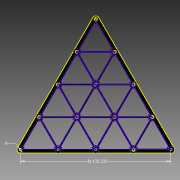
# Autodesk Inventor part: g16-bezel
Saved by Autodesk Inventor 2013 (Build 170138000, 138)
## iProperties
Created: 2013-03-21
Part Number: g16-bezel
Material: Acrylic
Document SubType Name: Modeling
Designer: TechShop Member
Density: 1 g/cm^3
d2: 6.000 mm
d5: 3.000 mm
Bolt_HeadDiameter: 6.000 mm
Bolt_HoleDiameter: 3.000 mm
LayerThickness: 2.750 mm
Pixel_BorderWidth: 1.000 mm
Pixel_Stride: 33.333 mm
Base_SideWidth: 133.332 mm
d24: 6.000 mm
d4: 0.00 deg
Author: TechShop Member
Autodesk Inventor part; units mm, degrees
(part 1 of 2)
ref_plane "YZ Plane" through (0, 0, 0) normal (1, 0, 0) x (0, 1, 0)
ref_plane "XZ Plane" through (0, 0, 0) normal (0, 1, 0) x (-1, 0, 0)
ref_plane "XY Plane" through (0, 0, 0) normal (0, 0, 1) x (1, 0, 0)
sketch "Triangle Hole Template" plane through (0, 0, 0) normal (0, 0, 1) x (1, 0, 0)
  line L0 (-99.9974, -57.7156) -> (-66.6644, -57.7156) construction
  line L1 (-66.6644, -57.7156) -> (-83.3309, -86.5829) construction
  line L2 (-83.3309, -86.5829) -> (-99.9974, -57.7156) construction
  line L3 (-99.1314, -58.2156) -> (-67.5304, -58.2156) construction
  line L4 (-67.5304, -58.2156) -> (-83.3309, -85.5829) construction
  line L5 (-83.3309, -85.5829) -> (-99.1314, -58.2156) construction
  line L6 (-83.3309, -58.2156) -> (-83.3309, -57.7156) construction
  line L7 (-75.4307, -71.8992) -> (-74.9976, -72.1492) construction
  line L8 (-91.2311, -71.8992) -> (-91.6641, -72.1492) construction
  arc A0 (-68.5696, -60.0156) -> (-69.6089, -58.2156) centre (-69.6089, -59.4156) ccw
  arc A1 (-84.3701, -83.7829) -> (-82.2917, -83.7829) centre (-83.3309, -83.1829) ccw
  arc A2 (-97.0529, -58.2156) -> (-98.0921, -60.0156) centre (-97.0529, -59.4156) ccw
  line L9 (-97.0529, -58.2156) -> (-69.6089, -58.2156)
  line L10 (-68.5696, -60.0156) -> (-82.2917, -83.7829)
  line L11 (-84.3701, -83.7829) -> (-98.0921, -60.0156)
  circle A3 centre (-98.4385, -58.6156) radius 0.4 construction
  line L12 (-98.0921, -58.8156) -> (-98.785, -58.4156) construction
  circle A4 centre (-99.9974, -57.7156) radius 3 construction
  line L13 (-83.3309, -57.7156) -> (-83.3309, -57.2156) construction
  line L14 (-98.0921, -58.8156) -> (-97.3993, -59.2156) construction
  point P0 (-85.6081, -66.0431)
  dimension "d24" = 6
  dimension "Pixel_BorderWidth" = 1
  dimension "Pixel_Stride" = 33.333
  measures "Pixel_BorderWidth" distance of L13.end L6.start
  measures "Pixel_Stride" distance of L0.start L0.end
sketch "Triangle Hole Template x16" plane through (0, 0, 0) normal (0, 0, 1) x (1, 0, 0)
  line L0 (-99.9974, -57.7156) -> (-66.6644, -57.7156) construction
  line L1 (-66.6644, -57.7156) -> (-83.3309, -86.5829) construction
  line L2 (-83.3309, -86.5829) -> (-99.9974, -57.7156) construction
  line L3 (-99.1314, -58.2156) -> (-67.5304, -58.2156) construction
  line L4 (-67.5304, -58.2156) -> (-83.3309, -85.5829) construction
  line L5 (-83.3309, -85.5829) -> (-99.1314, -58.2156) construction
  line L6 (-83.3309, -58.2156) -> (-83.3309, -57.7156) construction
  line L7 (-75.4307, -71.8992) -> (-74.9976, -72.1492) construction
  line L8 (-91.2311, -71.8992) -> (-91.6641, -72.1492) construction
  arc A0 (-68.5696, -60.0156) -> (-69.6089, -58.2156) centre (-69.6089, -59.4156) ccw
  arc A1 (-84.3701, -83.7829) -> (-82.2917, -83.7829) centre (-83.3309, -83.1829) ccw
  arc A2 (-97.0529, -58.2156) -> (-98.0921, -60.0156) centre (-97.0529, -59.4156) ccw
  line L9 (-97.0529, -58.2156) -> (-69.6089, -58.2156)
  line L10 (-68.5696, -60.0156) -> (-82.2917, -83.7829)
  line L11 (-84.3701, -83.7829) -> (-98.0921, -60.0156)
  circle A3 centre (-98.4385, -58.6156) radius 0.4 construction
  line L12 (-98.0921, -58.8156) -> (-98.785, -58.4156) construction
  circle A4 centre (-99.9974, -57.7156) radius 3 construction
  line L13 (-83.3309, -57.7156) -> (-83.3309, -57.2156) construction
  line L14 (-98.0921, -58.8156) -> (-97.3993, -59.2156) construction
  line L15 (-83.3309, -86.5829) -> (-49.9979, -86.5829) construction
  line L16 (-49.9979, -86.5829) -> (-66.6644, -115.4501) construction
  line L17 (-66.6644, -115.4501) -> (-83.3309, -86.5829) construction
  line L18 (-82.4649, -87.0829) -> (-50.8639, -87.0829) construction
  line L19 (-50.8639, -87.0829) -> (-66.6644, -114.4501) construction
  line L20 (-66.6644, -114.4501) -> (-82.4649, -87.0829) construction
  line L21 (-66.6644, -87.0829) -> (-66.6644, -86.5829) construction
  line L22 (-58.7642, -100.7665) -> (-58.3311, -101.0165) construction
  line L23 (-74.5646, -100.7665) -> (-74.9976, -101.0165) construction
  arc A5 (-51.9031, -88.8829) -> (-52.9424, -87.0829) centre (-52.9424, -88.2829) ccw
  arc A6 (-67.7036, -112.6501) -> (-65.6252, -112.6501) centre (-66.6644, -112.0501) ccw
  arc A7 (-80.3864, -87.0829) -> (-81.4256, -88.8829) centre (-80.3864, -88.2829) ccw
  line L24 (-80.3864, -87.0829) -> (-52.9424, -87.0829)
  line L25 (-51.9031, -88.8829) -> (-65.6252, -112.6501)
  line L26 (-67.7036, -112.6501) -> (-81.4256, -88.8829)
  circle A8 centre (-81.772, -87.4829) radius 0.4 construction
  line L27 (-81.4256, -87.6829) -> (-82.1185, -87.2829) construction
  circle A9 centre (-83.3309, -86.5829) radius 3 construction
  line L28 (-66.6644, -86.5829) -> (-66.6644, -86.0829) construction
  line L29 (-81.4256, -87.6829) -> (-80.7328, -88.0829) construction
  line L30 (-66.6676, -57.7533) -> (-33.3346, -57.7533) construction
  line L31 (-33.3346, -57.7533) -> (-50.0011, -86.6205) construction
  line L32 (-50.0011, -86.6205) -> (-66.6676, -57.7533) construction
  line L33 (-65.8016, -58.2533) -> (-34.2006, -58.2533) construction
  line L34 (-34.2006, -58.2533) -> (-50.0011, -85.6205) construction
  line L35 (-50.0011, -85.6205) -> (-65.8016, -58.2533) construction
  line L36 (-50.0011, -58.2533) -> (-50.0011, -57.7533) construction
  line L37 (-42.1009, -71.9369) -> (-41.6679, -72.1869) construction
  line L38 (-57.9013, -71.9369) -> (-58.3344, -72.1869) construction
  arc A10 (-35.2399, -60.0533) -> (-36.2791, -58.2533) centre (-36.2791, -59.4533) ccw
  arc A11 (-51.0403, -83.8205) -> (-48.9619, -83.8205) centre (-50.0011, -83.2205) ccw
  arc A12 (-63.7231, -58.2533) -> (-64.7624, -60.0533) centre (-63.7231, -59.4533) ccw
  line L39 (-63.7231, -58.2533) -> (-36.2791, -58.2533)
  line L40 (-35.2399, -60.0533) -> (-48.9619, -83.8205)
  line L41 (-51.0403, -83.8205) -> (-64.7624, -60.0533)
  circle A13 centre (-65.1088, -58.6533) radius 0.4 construction
  line L42 (-64.7624, -58.8533) -> (-65.4552, -58.4533) construction
  circle A14 centre (-66.6676, -57.7533) radius 3 construction
  line L43 (-50.0011, -57.7533) -> (-50.0011, -57.2533) construction
  line L44 (-64.7624, -58.8533) -> (-64.0695, -59.2533) construction
  line L45 (-50.0011, -86.6205) -> (-83.3341, -86.6205) construction
  line L46 (-83.3341, -86.6205) -> (-66.6676, -57.7533) construction
  line L47 (-66.6676, -57.7533) -> (-50.0011, -86.6205) construction
  line L48 (-50.8671, -86.1205) -> (-82.4681, -86.1205) construction
  line L49 (-82.4681, -86.1205) -> (-66.6676, -58.7533) construction
  line L50 (-66.6676, -58.7533) -> (-50.8671, -86.1205) construction
  line L51 (-66.6676, -86.1205) -> (-66.6676, -86.6205) construction
  line L52 (-74.5678, -72.4369) -> (-75.0009, -72.1869) construction
  line L53 (-58.7674, -72.4369) -> (-58.3344, -72.1869) construction
  arc A15 (-81.4289, -84.3205) -> (-80.3896, -86.1205) centre (-80.3896, -84.9205) ccw
  arc A16 (-65.6284, -60.5533) -> (-67.7068, -60.5533) centre (-66.6676, -61.1533) ccw
  arc A17 (-52.9456, -86.1205) -> (-51.9064, -84.3205) centre (-52.9456, -84.9205) ccw
  line L54 (-52.9456, -86.1205) -> (-80.3896, -86.1205)
  line L55 (-81.4289, -84.3205) -> (-67.7068, -60.5533)
  line L56 (-65.6284, -60.5533) -> (-51.9064, -84.3205)
  circle A18 centre (-51.56, -85.7205) radius 0.4 construction
  line L57 (-51.9064, -85.5205) -> (-51.2135, -85.9205) construction
  circle A19 centre (-50.0011, -86.6205) radius 3 construction
  line L58 (-66.6676, -86.6205) -> (-66.6676, -87.1205) construction
  line L59 (-51.9064, -85.5205) -> (-52.5992, -85.1205) construction
  line L60 (-33.3346, -57.7533) -> (-66.6676, -57.7533) construction
  line L61 (-66.6676, -57.7533) -> (-50.0011, -28.886) construction
  line L62 (-50.0011, -28.886) -> (-33.3346, -57.7533) construction
  line L63 (-34.2006, -57.2533) -> (-65.8016, -57.2533) construction
  line L64 (-65.8016, -57.2533) -> (-50.0011, -29.886) construction
  line L65 (-50.0011, -29.886) -> (-34.2006, -57.2533) construction
  line L66 (-50.0011, -57.2533) -> (-50.0011, -57.7533) construction
  line L67 (-57.9013, -43.5697) -> (-58.3344, -43.3197) construction
  line L68 (-42.1009, -43.5697) -> (-41.6679, -43.3197) construction
  arc A20 (-64.7624, -55.4533) -> (-63.7231, -57.2533) centre (-63.7231, -56.0533) ccw
  arc A21 (-48.9619, -31.686) -> (-51.0403, -31.686) centre (-50.0011, -32.286) ccw
  arc A22 (-36.2791, -57.2533) -> (-35.2399, -55.4533) centre (-36.2791, -56.0533) ccw
  line L69 (-36.2791, -57.2533) -> (-63.7231, -57.2533)
  line L70 (-64.7624, -55.4533) -> (-51.0403, -31.686)
  line L71 (-48.9619, -31.686) -> (-35.2399, -55.4533)
  circle A23 centre (-34.8935, -56.8533) radius 0.4 construction
  line L72 (-35.2399, -56.6533) -> (-34.547, -57.0533) construction
  circle A24 centre (-33.3346, -57.7533) radius 3 construction
  line L73 (-50.0011, -57.7533) -> (-50.0011, -58.2533) construction
  line L74 (-35.2399, -56.6533) -> (-35.9327, -56.2533) construction
  line L75 (-66.6676, -57.7156) -> (-100.0006, -57.7156) construction
  line L76 (-100.0006, -57.7156) -> (-83.3341, -28.8484) construction
  line L77 (-83.3341, -28.8484) -> (-66.6676, -57.7156) construction
  line L78 (-67.5336, -57.2156) -> (-99.1346, -57.2156) construction
  line L79 (-99.1346, -57.2156) -> (-83.3341, -29.8484) construction
  line L80 (-83.3341, -29.8484) -> (-67.5336, -57.2156) construction
  line L81 (-83.3341, -57.2156) -> (-83.3341, -57.7156) construction
  line L82 (-91.2343, -43.532) -> (-91.6674, -43.282) construction
  line L83 (-75.4339, -43.532) -> (-75.0009, -43.282) construction
  arc A25 (-98.0954, -55.4156) -> (-97.0561, -57.2156) centre (-97.0561, -56.0156) ccw
  arc A26 (-82.2949, -31.6484) -> (-84.3733, -31.6484) centre (-83.3341, -32.2484) ccw
  arc A27 (-69.6121, -57.2156) -> (-68.5729, -55.4156) centre (-69.6121, -56.0156) ccw
  line L84 (-69.6121, -57.2156) -> (-97.0561, -57.2156)
  line L85 (-98.0954, -55.4156) -> (-84.3733, -31.6484)
  line L86 (-82.2949, -31.6484) -> (-68.5729, -55.4156)
  circle A28 centre (-68.2265, -56.8156) radius 0.4 construction
  line L87 (-68.5729, -56.6156) -> (-67.88, -57.0156) construction
  circle A29 centre (-66.6676, -57.7156) radius 3 construction
  line L88 (-83.3341, -57.7156) -> (-83.3341, -58.2156) construction
  line L89 (-68.5729, -56.6156) -> (-69.2657, -56.2156) construction
  line L90 (-83.3186, -28.8752) -> (-116.6516, -28.8752) construction
  line L91 (-116.6516, -28.8752) -> (-99.9851, -0.008) construction
  line L92 (-99.9851, -0.008) -> (-83.3186, -28.8752) construction
  line L93 (-84.1846, -28.3752) -> (-115.7856, -28.3752) construction
  line L94 (-115.7856, -28.3752) -> (-99.9851, -1.008) construction
  line L95 (-99.9851, -1.008) -> (-84.1846, -28.3752) construction
  line L96 (-99.9851, -28.3752) -> (-99.9851, -28.8752) construction
  line L97 (-107.8853, -14.6916) -> (-108.3184, -14.4416) construction
  line L98 (-92.0849, -14.6916) -> (-91.6519, -14.4416) construction
  arc A30 (-114.7464, -26.5752) -> (-113.7071, -28.3752) centre (-113.7071, -27.1752) ccw
  arc A31 (-98.9459, -2.808) -> (-101.0243, -2.808) centre (-99.9851, -3.408) ccw
  arc A32 (-86.2631, -28.3752) -> (-85.2239, -26.5752) centre (-86.2631, -27.1752) ccw
  line L99 (-86.2631, -28.3752) -> (-113.7071, -28.3752)
  line L100 (-114.7464, -26.5752) -> (-101.0243, -2.808)
  line L101 (-98.9459, -2.808) -> (-85.2239, -26.5752)
  circle A33 centre (-84.8775, -27.9752) radius 0.4 construction
  line L102 (-85.2239, -27.7752) -> (-84.531, -28.1752) construction
  circle A34 centre (-83.3186, -28.8752) radius 3 construction
  line L103 (-99.9851, -28.8752) -> (-99.9851, -29.3752) construction
  line L104 (-85.2239, -27.7752) -> (-85.9167, -27.3752) construction
  line L105 (-50.0011, -28.8484) -> (-83.3341, -28.8484) construction
  line L106 (-83.3341, -28.8484) -> (-66.6676, 0.0188) construction
  line L107 (-66.6676, 0.0188) -> (-50.0011, -28.8484) construction
  line L108 (-50.8671, -28.3484) -> (-82.4681, -28.3484) construction
  line L109 (-82.4681, -28.3484) -> (-66.6676, -0.9812) construction
  line L110 (-66.6676, -0.9812) -> (-50.8671, -28.3484) construction
  line L111 (-66.6676, -28.3484) -> (-66.6676, -28.8484) construction
  line L112 (-74.5678, -14.6648) -> (-75.0009, -14.4148) construction
  line L113 (-58.7674, -14.6648) -> (-58.3344, -14.4148) construction
  arc A35 (-81.4289, -26.5484) -> (-80.3896, -28.3484) centre (-80.3896, -27.1484) ccw
  arc A36 (-65.6284, -2.7812) -> (-67.7068, -2.7812) centre (-66.6676, -3.3812) ccw
  arc A37 (-52.9456, -28.3484) -> (-51.9064, -26.5484) centre (-52.9456, -27.1484) ccw
  line L114 (-52.9456, -28.3484) -> (-80.3896, -28.3484)
  line L115 (-81.4289, -26.5484) -> (-67.7068, -2.7812)
  line L116 (-65.6284, -2.7812) -> (-51.9064, -26.5484)
  circle A38 centre (-51.56, -27.9484) radius 0.4 construction
  line L117 (-51.9064, -27.7484) -> (-51.2135, -28.1484) construction
  circle A39 centre (-50.0011, -28.8484) radius 3 construction
  line L118 (-66.6676, -28.8484) -> (-66.6676, -29.3484) construction
  line L119 (-51.9064, -27.7484) -> (-52.5992, -27.3484) construction
  line L120 (-16.6681, -28.8484) -> (-50.0011, -28.8484) construction
  line L121 (-50.0011, -28.8484) -> (-33.3346, 0.0188) construction
  line L122 (-33.3346, 0.0188) -> (-16.6681, -28.8484) construction
  line L123 (-17.5341, -28.3484) -> (-49.1351, -28.3484) construction
  line L124 (-49.1351, -28.3484) -> (-33.3346, -0.9812) construction
  line L125 (-33.3346, -0.9812) -> (-17.5341, -28.3484) construction
  line L126 (-33.3346, -28.3484) -> (-33.3346, -28.8484) construction
  line L127 (-41.2348, -14.6648) -> (-41.6679, -14.4148) construction
  line L128 (-25.4344, -14.6648) -> (-25.0014, -14.4148) construction
  arc A40 (-48.0959, -26.5484) -> (-47.0566, -28.3484) centre (-47.0566, -27.1484) ccw
  arc A41 (-32.2954, -2.7812) -> (-34.3738, -2.7812) centre (-33.3346, -3.3812) ccw
  arc A42 (-19.6126, -28.3484) -> (-18.5734, -26.5484) centre (-19.6126, -27.1484) ccw
  line L129 (-19.6126, -28.3484) -> (-47.0566, -28.3484)
  line L130 (-48.0959, -26.5484) -> (-34.3738, -2.7812)
  line L131 (-32.2954, -2.7812) -> (-18.5734, -26.5484)
  circle A43 centre (-18.227, -27.9484) radius 0.4 construction
  line L132 (-18.5734, -27.7484) -> (-17.8805, -28.1484) construction
  circle A44 centre (-16.6681, -28.8484) radius 3 construction
  line L133 (-33.3346, -28.8484) -> (-33.3346, -29.3484) construction
  line L134 (-18.5734, -27.7484) -> (-19.2662, -27.3484) construction
  line L135 (-49.9979, -28.8484) -> (-16.6649, -28.8484) construction
  line L136 (-16.6649, -28.8484) -> (-33.3314, -57.7156) construction
  line L137 (-33.3314, -57.7156) -> (-49.9979, -28.8484) construction
  line L138 (-49.1319, -29.3484) -> (-17.5309, -29.3484) construction
  line L139 (-17.5309, -29.3484) -> (-33.3314, -56.7156) construction
  line L140 (-33.3314, -56.7156) -> (-49.1319, -29.3484) construction
  line L141 (-33.3314, -29.3484) -> (-33.3314, -28.8484) construction
  line L142 (-25.4312, -43.032) -> (-24.9981, -43.282) construction
  line L143 (-41.2316, -43.032) -> (-41.6646, -43.282) construction
  arc A45 (-18.5701, -31.1484) -> (-19.6094, -29.3484) centre (-19.6094, -30.5484) ccw
  arc A46 (-34.3706, -54.9156) -> (-32.2922, -54.9156) centre (-33.3314, -54.3156) ccw
  arc A47 (-47.0534, -29.3484) -> (-48.0926, -31.1484) centre (-47.0534, -30.5484) ccw
  line L144 (-47.0534, -29.3484) -> (-19.6094, -29.3484)
  line L145 (-18.5701, -31.1484) -> (-32.2922, -54.9156)
  line L146 (-34.3706, -54.9156) -> (-48.0926, -31.1484)
  circle A48 centre (-48.439, -29.7484) radius 0.4 construction
  line L147 (-48.0926, -29.9484) -> (-48.7855, -29.5484) construction
  circle A49 centre (-49.9979, -28.8484) radius 3 construction
  line L148 (-33.3314, -28.8484) -> (-33.3314, -28.3484) construction
  line L149 (-48.0926, -29.9484) -> (-47.3998, -30.3484) construction
  line L150 (-66.6676, 0.0188) -> (-33.3346, 0.0188) construction
  line L151 (-33.3346, 0.0188) -> (-50.0011, -28.8484) construction
  line L152 (-50.0011, -28.8484) -> (-66.6676, 0.0188) construction
  line L153 (-65.8016, -0.4812) -> (-34.2006, -0.4812) construction
  line L154 (-34.2006, -0.4812) -> (-50.0011, -27.8484) construction
  line L155 (-50.0011, -27.8484) -> (-65.8016, -0.4812) construction
  line L156 (-50.0011, -0.4812) -> (-50.0011, 0.0188) construction
  line L157 (-42.1009, -14.1648) -> (-41.6679, -14.4148) construction
  line L158 (-57.9013, -14.1648) -> (-58.3344, -14.4148) construction
  arc A50 (-35.2399, -2.2812) -> (-36.2791, -0.4812) centre (-36.2791, -1.6812) ccw
  arc A51 (-51.0403, -26.0484) -> (-48.9619, -26.0484) centre (-50.0011, -25.4484) ccw
  arc A52 (-63.7231, -0.4812) -> (-64.7624, -2.2812) centre (-63.7231, -1.6812) ccw
  line L159 (-63.7231, -0.4812) -> (-36.2791, -0.4812)
  line L160 (-35.2399, -2.2812) -> (-48.9619, -26.0484)
  line L161 (-51.0403, -26.0484) -> (-64.7624, -2.2812)
  circle A53 centre (-65.1088, -0.8812) radius 0.4 construction
  line L162 (-64.7624, -1.0812) -> (-65.4552, -0.6812) construction
  circle A54 centre (-66.6676, 0.0188) radius 3 construction
  line L163 (-50.0011, 0.0188) -> (-50.0011, 0.5188) construction
  line L164 (-64.7624, -1.0812) -> (-64.0695, -1.4812) construction
  line L165 (-33.3314, 0.0188) -> (0.0016, 0.0188) construction
  line L166 (0.0016, 0.0188) -> (-16.6649, -28.8484) construction
  line L167 (-16.6649, -28.8484) -> (-33.3314, 0.0188) construction
  line L168 (-32.4654, -0.4812) -> (-0.8644, -0.4812) construction
  line L169 (-0.8644, -0.4812) -> (-16.6649, -27.8484) construction
  line L170 (-16.6649, -27.8484) -> (-32.4654, -0.4812) construction
  line L171 (-16.6649, -0.4812) -> (-16.6649, 0.0188) construction
  line L172 (-8.7647, -14.1648) -> (-8.3316, -14.4148) construction
  line L173 (-24.5651, -14.1648) -> (-24.9981, -14.4148) construction
  arc A55 (-1.9036, -2.2812) -> (-2.9429, -0.4812) centre (-2.9429, -1.6812) ccw
  arc A56 (-17.7041, -26.0484) -> (-15.6257, -26.0484) centre (-16.6649, -25.4484) ccw
  arc A57 (-30.3869, -0.4812) -> (-31.4261, -2.2812) centre (-30.3869, -1.6812) ccw
  line L174 (-30.3869, -0.4812) -> (-2.9429, -0.4812)
  line L175 (-1.9036, -2.2812) -> (-15.6257, -26.0484)
  line L176 (-17.7041, -26.0484) -> (-31.4261, -2.2812)
  circle A58 centre (-31.7725, -0.8812) radius 0.4 construction
  line L177 (-31.4261, -1.0812) -> (-32.119, -0.6812) construction
  circle A59 centre (-33.3314, 0.0188) radius 3 construction
  line L178 (-16.6649, 0.0188) -> (-16.6649, 0.5188) construction
  line L179 (-31.4261, -1.0812) -> (-30.7333, -1.4812) construction
  line L180 (-83.317, -28.8188) -> (-49.984, -28.8188) construction
  line L181 (-49.984, -28.8188) -> (-66.6505, -57.686) construction
  line L182 (-66.6505, -57.686) -> (-83.317, -28.8188) construction
  line L183 (-82.451, -29.3188) -> (-50.85, -29.3188) construction
  line L184 (-50.85, -29.3188) -> (-66.6505, -56.686) construction
  line L185 (-66.6505, -56.686) -> (-82.451, -29.3188) construction
  line L186 (-66.6505, -29.3188) -> (-66.6505, -28.8188) construction
  line L187 (-58.7503, -43.0024) -> (-58.3173, -43.2524) construction
  line L188 (-74.5507, -43.0024) -> (-74.9838, -43.2524) construction
  arc A60 (-51.8893, -31.1188) -> (-52.9285, -29.3188) centre (-52.9285, -30.5188) ccw
  arc A61 (-67.6897, -54.886) -> (-65.6113, -54.886) centre (-66.6505, -54.286) ccw
  arc A62 (-80.3725, -29.3188) -> (-81.4117, -31.1188) centre (-80.3725, -30.5188) ccw
  line L189 (-80.3725, -29.3188) -> (-52.9285, -29.3188)
  line L190 (-51.8893, -31.1188) -> (-65.6113, -54.886)
  line L191 (-67.6897, -54.886) -> (-81.4117, -31.1188)
  circle A63 centre (-81.7582, -29.7188) radius 0.4 construction
  line L192 (-81.4117, -29.9188) -> (-82.1046, -29.5188) construction
  circle A64 centre (-83.317, -28.8188) radius 3 construction
  line L193 (-66.6505, -28.8188) -> (-66.6505, -28.3188) construction
  line L194 (-81.4117, -29.9188) -> (-80.7189, -30.3188) construction
  line L195 (-99.9974, 0.0188) -> (-66.6644, 0.0188) construction
  line L196 (-66.6644, 0.0188) -> (-83.3309, -28.8484) construction
  line L197 (-83.3309, -28.8484) -> (-99.9974, 0.0188) construction
  line L198 (-99.1314, -0.4812) -> (-67.5304, -0.4812) construction
  line L199 (-67.5304, -0.4812) -> (-83.3309, -27.8484) construction
  line L200 (-83.3309, -27.8484) -> (-99.1314, -0.4812) construction
  line L201 (-83.3309, -0.4812) -> (-83.3309, 0.0188) construction
  line L202 (-75.4307, -14.1648) -> (-74.9976, -14.4148) construction
  line L203 (-91.2311, -14.1648) -> (-91.6641, -14.4148) construction
  arc A65 (-68.5696, -2.2812) -> (-69.6089, -0.4812) centre (-69.6089, -1.6812) ccw
  arc A66 (-84.3701, -26.0484) -> (-82.2917, -26.0484) centre (-83.3309, -25.4484) ccw
  arc A67 (-97.0529, -0.4812) -> (-98.0921, -2.2812) centre (-97.0529, -1.6812) ccw
  line L204 (-97.0529, -0.4812) -> (-69.6089, -0.4812)
  line L205 (-68.5696, -2.2812) -> (-82.2917, -26.0484)
  line L206 (-84.3701, -26.0484) -> (-98.0921, -2.2812)
  circle A68 centre (-98.4385, -0.8812) radius 0.4 construction
  line L207 (-98.0921, -1.0812) -> (-98.785, -0.6812) construction
  circle A69 centre (-99.9974, 0.0188) radius 3 construction
  line L208 (-83.3309, 0.0188) -> (-83.3309, 0.5188) construction
  line L209 (-98.0921, -1.0812) -> (-97.3993, -1.4812) construction
  line L210 (-133.3304, -0.008) -> (-99.9974, -0.008) construction
  line L211 (-99.9974, -0.008) -> (-116.6639, -28.8752) construction
  line L212 (-116.6639, -28.8752) -> (-133.3304, -0.008) construction
  line L213 (-132.4644, -0.508) -> (-100.8634, -0.508) construction
  line L214 (-100.8634, -0.508) -> (-116.6639, -27.8752) construction
  line L215 (-116.6639, -27.8752) -> (-132.4644, -0.508) construction
  line L216 (-116.6639, -0.508) -> (-116.6639, -0.008) construction
  line L217 (-108.7637, -14.1916) -> (-108.3306, -14.4416) construction
  line L218 (-124.5641, -14.1916) -> (-124.9971, -14.4416) construction
  arc A70 (-101.9026, -2.308) -> (-102.9419, -0.508) centre (-102.9419, -1.708) ccw
  arc A71 (-117.7031, -26.0752) -> (-115.6247, -26.0752) centre (-116.6639, -25.4752) ccw
  arc A72 (-130.3859, -0.508) -> (-131.4251, -2.308) centre (-130.3859, -1.708) ccw
  line L219 (-130.3859, -0.508) -> (-102.9419, -0.508)
  line L220 (-101.9026, -2.308) -> (-115.6247, -26.0752)
  line L221 (-117.7031, -26.0752) -> (-131.4251, -2.308)
  circle A73 centre (-131.7715, -0.908) radius 0.4 construction
  line L222 (-131.4251, -1.108) -> (-132.118, -0.708) construction
  circle A74 centre (-133.3304, -0.008) radius 3 construction
  line L223 (-116.6639, -0.008) -> (-116.6639, 0.492) construction
  line L224 (-131.4251, -1.108) -> (-130.7323, -1.508) construction
  line L225 (-116.6671, -28.8484) -> (-83.3341, -28.8484) construction
  line L226 (-83.3341, -28.8484) -> (-100.0006, -57.7156) construction
  line L227 (-100.0006, -57.7156) -> (-116.6671, -28.8484) construction
  line L228 (-115.8011, -29.3484) -> (-84.2001, -29.3484) construction
  line L229 (-84.2001, -29.3484) -> (-100.0006, -56.7156) construction
  line L230 (-100.0006, -56.7156) -> (-115.8011, -29.3484) construction
  line L231 (-100.0006, -29.3484) -> (-100.0006, -28.8484) construction
  line L232 (-92.1004, -43.032) -> (-91.6674, -43.282) construction
  line L233 (-107.9008, -43.032) -> (-108.3339, -43.282) construction
  arc A75 (-85.2394, -31.1484) -> (-86.2786, -29.3484) centre (-86.2786, -30.5484) ccw
  arc A76 (-101.0398, -54.9156) -> (-98.9614, -54.9156) centre (-100.0006, -54.3156) ccw
  arc A77 (-113.7226, -29.3484) -> (-114.7619, -31.1484) centre (-113.7226, -30.5484) ccw
  line L234 (-113.7226, -29.3484) -> (-86.2786, -29.3484)
  line L235 (-85.2394, -31.1484) -> (-98.9614, -54.9156)
  line L236 (-101.0398, -54.9156) -> (-114.7619, -31.1484)
  circle A78 centre (-115.1083, -29.7484) radius 0.4 construction
  line L237 (-114.7619, -29.9484) -> (-115.4547, -29.5484) construction
  circle A79 centre (-116.6671, -28.8484) radius 3 construction
  line L238 (-100.0006, -28.8484) -> (-100.0006, -28.3484) construction
  line L239 (-114.7619, -29.9484) -> (-114.069, -30.3484) construction
  point P0 (-67.2349, -38.1612)
sketch "Border Sketch" plane through (0, 0, 0) normal (0, 1, 0) x (-1, 0, 0)
  line L0 (0, 0) -> (133.332, 0) construction
  line L1 (0, 0) -> (66.666, 115.4689) construction
  line L2 (66.666, 115.4689) -> (133.332, 0) construction
  circle A0 centre (0, 0) radius 3 construction
  circle A1 centre (66.666, 115.4689) radius 3 construction
  circle A2 centre (133.332, 0) radius 3 construction
  line L3 (69.2641, 116.9689) -> (135.9301, 1.5)
  arc A3 (69.2641, 116.9689) -> (64.0679, 116.9689) centre (66.666, 115.4689) ccw
  arc A4 (133.332, -3) -> (135.9301, 1.5) centre (133.332, 0) ccw
  arc A5 (-2.5981, 1.5) -> (0, -3) centre (0, 0) ccw
  line L4 (0, -3) -> (133.332, -3)
  line L5 (-2.5981, 1.5) -> (64.0679, 116.9689)
  dimension "Bolt_HeadDiameter" = 6
  dimension "Base_SideWidth" = 133.332
  constraints: 12 end point, 12 point on circle, 11 tangent, 6 centre point, 4 coincident, 2 equal length, 2 equal radius, 1 horizontal, 1 parallel
  measures "Bolt_HeadDiameter" diameter of A0
  measures "Base_SideWidth" distance of L0.start L0.end
extrude "Border" add sketch "Border Sketch" along normal blind 2.75
sketch "Bolt Hole Sketch" plane through (0, 2.75, 0) normal (0, 1, 0) x (1, 0, 0)
  arc A0 (-69.2641, -116.9689) -> (-64.0679, -116.9689) centre (-66.666, -115.4689) ccw projected
  arc A1 (2.5981, -1.5) -> (0, 3) centre (0, 0) ccw projected
  arc A2 (-133.332, 3) -> (-135.9301, -1.5) centre (-133.332, 0) ccw projected
  line L0 (-135.9301, -1.5) -> (-69.2641, -116.9689) projected
  line L1 (-64.0679, -116.9689) -> (2.5981, -1.5) projected
  line L2 (0, 3) -> (-133.332, 3) projected
  line L3 (-66.666, -115.4689) -> (0, 0) construction
  line L4 (0, 0) -> (-133.332, 0) construction
  line L5 (-133.332, 0) -> (-66.666, -115.4689) construction
  line L6 (-99.999, -57.7344) -> (-33.333, -57.7344) construction
  line L7 (-33.333, -57.7344) -> (-66.666, 0) construction
  line L8 (-99.999, -57.7344) -> (-66.666, 0) construction
  line L9 (-49.9995, -28.8672) -> (-33.333, 0) construction
  line L10 (-33.333, 0) -> (-16.6665, -28.8672) construction
  line L11 (-16.6665, -28.8672) -> (-116.6655, -28.8672) construction
  line L12 (-116.6655, -28.8672) -> (-99.999, 0) construction
  line L13 (-49.9995, -28.8672) -> (-83.3325, -86.6017) construction
  line L14 (-49.9995, -86.6017) -> (-83.3325, -86.6017) construction
  line L15 (-49.9995, -86.6017) -> (-66.666, -57.7344) construction
  line L16 (-66.666, -57.7344) -> (-83.3325, -28.8672) construction
  line L17 (-83.3325, -28.8672) -> (-99.999, 0) construction
  constraints: 30 end point, 10 parallel, 7 point on line, 6 midpoint, 1 collinear
hole "Bolt Holes" at (-133.332, 2.75, 0) at (0, 2.75, 0) at (-66.666, 2.75, 115.4689) at (-99.999, 2.75, 0) at (-116.6655, 2.75, 28.8672) at (-66.666, 2.75, 0) at (-49.9995, 2.75, 28.8672) at (-33.333, 2.75, 0) at (-16.6665, 2.75, 28.8672) at (-33.333, 2.75, 57.7344) at (-49.9995, 2.75, 86.6017) at (-83.3325, 2.75, 86.6017) at (-99.999, 2.75, 57.7344) at (-66.666, 2.75, 57.7344) at (-83.3325, 2.75, 28.8672) direction (0, -1, 0) diameter 3 end through all
sketch "Pixel Hole Sketch" plane through (0, 2.75, 0) normal (0, 1, 0) x (1, 0, 0)
  circle A0 centre (-66.666, -57.7344) radius 1.5 projected
  circle A1 centre (-83.3325, -86.6017) radius 1.5 projected
  circle A2 centre (-33.333, -57.7344) radius 1.5 projected
  circle A3 centre (-99.999, 0) radius 1.5 projected
  circle A4 centre (-66.666, -115.4689) radius 1.5 projected
  circle A5 centre (-116.6655, -28.8672) radius 1.5 projected
  circle A6 centre (-49.9995, -28.8672) radius 1.5 projected
  circle A7 centre (-16.6665, -28.8672) radius 1.5 projected
  circle A8 centre (-49.9995, -86.6017) radius 1.5 projected
  circle A9 centre (-99.999, -57.7344) radius 1.5 projected
  circle A10 centre (-83.3325, -28.8672) radius 1.5 projected
  line L0 (-135.9301, -1.5) -> (-69.2641, -116.9689) projected
  line L1 (-64.0679, -116.9689) -> (2.5981, -1.5) projected
  line L2 (0, 3) -> (-133.332, 3) projected
  line L3 (-99.9974, -57.7156) -> (-66.6644, -57.7156) construction
  line L4 (-66.6644, -57.7156) -> (-83.3309, -86.5829) construction
  line L5 (-83.3309, -86.5829) -> (-99.9974, -57.7156) construction
  line L6 (-99.1314, -58.2156) -> (-67.5304, -58.2156) construction
  line L7 (-67.5304, -58.2156) -> (-83.3309, -85.5829) construction
  line L8 (-83.3309, -85.5829) -> (-99.1314, -58.2156) construction
  line L9 (-83.3309, -58.2156) -> (-83.3309, -57.7156) construction
  line L10 (-75.4307, -71.8992) -> (-74.9976, -72.1492) construction
  line L11 (-91.2311, -71.8992) -> (-91.6641, -72.1492) construction
  arc A11 (-68.5696, -60.0156) -> (-69.6089, -58.2156) centre (-69.6089, -59.4156) ccw
  arc A12 (-84.3701, -83.7829) -> (-82.2917, -83.7829) centre (-83.3309, -83.1829) ccw
  arc A13 (-97.0529, -58.2156) -> (-98.0921, -60.0156) centre (-97.0529, -59.4156) ccw
  line L12 (-97.0529, -58.2156) -> (-69.6089, -58.2156)
  line L13 (-68.5696, -60.0156) -> (-82.2917, -83.7829)
  line L14 (-84.3701, -83.7829) -> (-98.0921, -60.0156)
  circle A14 centre (-98.4385, -58.6156) radius 0.4 construction
  line L15 (-98.0921, -58.8156) -> (-98.785, -58.4156) construction
  circle A15 centre (-99.9974, -57.7156) radius 3 construction
  line L16 (-83.3309, -57.7156) -> (-83.3309, -57.2156) construction
  line L17 (-98.0921, -58.8156) -> (-97.3993, -59.2156) construction
  line L18 (-83.3309, -86.5829) -> (-49.9979, -86.5829) construction
  line L19 (-49.9979, -86.5829) -> (-66.6644, -115.4501) construction
  line L20 (-66.6644, -115.4501) -> (-83.3309, -86.5829) construction
  line L21 (-82.4649, -87.0829) -> (-50.8639, -87.0829) construction
  line L22 (-50.8639, -87.0829) -> (-66.6644, -114.4501) construction
  line L23 (-66.6644, -114.4501) -> (-82.4649, -87.0829) construction
  line L24 (-66.6644, -87.0829) -> (-66.6644, -86.5829) construction
  line L25 (-58.7642, -100.7665) -> (-58.3311, -101.0165) construction
  line L26 (-74.5646, -100.7665) -> (-74.9976, -101.0165) construction
  arc A16 (-51.9031, -88.8829) -> (-52.9424, -87.0829) centre (-52.9424, -88.2829) ccw
  arc A17 (-67.7036, -112.6501) -> (-65.6252, -112.6501) centre (-66.6644, -112.0501) ccw
  arc A18 (-80.3864, -87.0829) -> (-81.4256, -88.8829) centre (-80.3864, -88.2829) ccw
  line L27 (-80.3864, -87.0829) -> (-52.9424, -87.0829)
  line L28 (-51.9031, -88.8829) -> (-65.6252, -112.6501)
  line L29 (-67.7036, -112.6501) -> (-81.4256, -88.8829)
  circle A19 centre (-81.772, -87.4829) radius 0.4 construction
  line L30 (-81.4256, -87.6829) -> (-82.1185, -87.2829) construction
  circle A20 centre (-83.3309, -86.5829) radius 3 construction
  line L31 (-66.6644, -86.5829) -> (-66.6644, -86.0829) construction
  line L32 (-81.4256, -87.6829) -> (-80.7328, -88.0829) construction
  line L33 (-66.6676, -57.7533) -> (-33.3346, -57.7533) construction
  line L34 (-33.3346, -57.7533) -> (-50.0011, -86.6205) construction
  line L35 (-50.0011, -86.6205) -> (-66.6676, -57.7533) construction
  line L36 (-65.8016, -58.2533) -> (-34.2006, -58.2533) construction
  line L37 (-34.2006, -58.2533) -> (-50.0011, -85.6205) construction
  line L38 (-50.0011, -85.6205) -> (-65.8016, -58.2533) construction
  line L39 (-50.0011, -58.2533) -> (-50.0011, -57.7533) construction
  line L40 (-42.1009, -71.9369) -> (-41.6679, -72.1869) construction
  line L41 (-57.9013, -71.9369) -> (-58.3344, -72.1869) construction
  arc A21 (-35.2399, -60.0533) -> (-36.2791, -58.2533) centre (-36.2791, -59.4533) ccw
  arc A22 (-51.0403, -83.8205) -> (-48.9619, -83.8205) centre (-50.0011, -83.2205) ccw
  arc A23 (-63.7231, -58.2533) -> (-64.7624, -60.0533) centre (-63.7231, -59.4533) ccw
  line L42 (-63.7231, -58.2533) -> (-36.2791, -58.2533)
  line L43 (-35.2399, -60.0533) -> (-48.9619, -83.8205)
  line L44 (-51.0403, -83.8205) -> (-64.7624, -60.0533)
  circle A24 centre (-65.1088, -58.6533) radius 0.4 construction
  line L45 (-64.7624, -58.8533) -> (-65.4552, -58.4533) construction
  circle A25 centre (-66.6676, -57.7533) radius 3 construction
  line L46 (-50.0011, -57.7533) -> (-50.0011, -57.2533) construction
  line L47 (-64.7624, -58.8533) -> (-64.0695, -59.2533) construction
  line L48 (-50.0011, -86.6205) -> (-83.3341, -86.6205) construction
  line L49 (-83.3341, -86.6205) -> (-66.6676, -57.7533) construction
  line L50 (-66.6676, -57.7533) -> (-50.0011, -86.6205) construction
  line L51 (-50.8671, -86.1205) -> (-82.4681, -86.1205) construction
  line L52 (-82.4681, -86.1205) -> (-66.6676, -58.7533) construction
  line L53 (-66.6676, -58.7533) -> (-50.8671, -86.1205) construction
  line L54 (-66.6676, -86.1205) -> (-66.6676, -86.6205) construction
  line L55 (-74.5678, -72.4369) -> (-75.0009, -72.1869) construction
  line L56 (-58.7674, -72.4369) -> (-58.3344, -72.1869) construction
  arc A26 (-81.4289, -84.3205) -> (-80.3896, -86.1205) centre (-80.3896, -84.9205) ccw
  arc A27 (-65.6284, -60.5533) -> (-67.7068, -60.5533) centre (-66.6676, -61.1533) ccw
  arc A28 (-52.9456, -86.1205) -> (-51.9064, -84.3205) centre (-52.9456, -84.9205) ccw
  line L57 (-52.9456, -86.1205) -> (-80.3896, -86.1205)
  line L58 (-81.4289, -84.3205) -> (-67.7068, -60.5533)
  line L59 (-65.6284, -60.5533) -> (-51.9064, -84.3205)
  circle A29 centre (-51.56, -85.7205) radius 0.4 construction
  line L60 (-51.9064, -85.5205) -> (-51.2135, -85.9205) construction
  circle A30 centre (-50.0011, -86.6205) radius 3 construction
  line L61 (-66.6676, -86.6205) -> (-66.6676, -87.1205) construction
  line L62 (-51.9064, -85.5205) -> (-52.5992, -85.1205) construction
  line L63 (-33.3346, -57.7533) -> (-66.6676, -57.7533) construction
  line L64 (-66.6676, -57.7533) -> (-50.0011, -28.886) construction
  line L65 (-50.0011, -28.886) -> (-33.3346, -57.7533) construction
  line L66 (-34.2006, -57.2533) -> (-65.8016, -57.2533) construction
  line L67 (-65.8016, -57.2533) -> (-50.0011, -29.886) construction
  line L68 (-50.0011, -29.886) -> (-34.2006, -57.2533) construction
  line L69 (-50.0011, -57.2533) -> (-50.0011, -57.7533) construction
  line L70 (-57.9013, -43.5697) -> (-58.3344, -43.3197) construction
  line L71 (-42.1009, -43.5697) -> (-41.6679, -43.3197) construction
  arc A31 (-64.7624, -55.4533) -> (-63.7231, -57.2533) centre (-63.7231, -56.0533) ccw
  arc A32 (-48.9619, -31.686) -> (-51.0403, -31.686) centre (-50.0011, -32.286) ccw
  arc A33 (-36.2791, -57.2533) -> (-35.2399, -55.4533) centre (-36.2791, -56.0533) ccw
  line L72 (-36.2791, -57.2533) -> (-63.7231, -57.2533)
  line L73 (-64.7624, -55.4533) -> (-51.0403, -31.686)
  line L74 (-48.9619, -31.686) -> (-35.2399, -55.4533)
  circle A34 centre (-34.8935, -56.8533) radius 0.4 construction
  line L75 (-35.2399, -56.6533) -> (-34.547, -57.0533) construction
  circle A35 centre (-33.3346, -57.7533) radius 3 construction
  line L76 (-50.0011, -57.7533) -> (-50.0011, -58.2533) construction
  line L77 (-35.2399, -56.6533) -> (-35.9327, -56.2533) construction
  line L78 (-66.6676, -57.7156) -> (-100.0006, -57.7156) construction
  line L79 (-100.0006, -57.7156) -> (-83.3341, -28.8484) construction
  line L80 (-83.3341, -28.8484) -> (-66.6676, -57.7156) construction
  line L81 (-67.5336, -57.2156) -> (-99.1346, -57.2156) construction
  line L82 (-99.1346, -57.2156) -> (-83.3341, -29.8484) construction
  line L83 (-83.3341, -29.8484) -> (-67.5336, -57.2156) construction
  line L84 (-83.3341, -57.2156) -> (-83.3341, -57.7156) construction
  line L85 (-91.2343, -43.532) -> (-91.6674, -43.282) construction
  line L86 (-75.4339, -43.532) -> (-75.0009, -43.282) construction
  arc A36 (-98.0954, -55.4156) -> (-97.0561, -57.2156) centre (-97.0561, -56.0156) ccw
  arc A37 (-82.2949, -31.6484) -> (-84.3733, -31.6484) centre (-83.3341, -32.2484) ccw
  arc A38 (-69.6121, -57.2156) -> (-68.5729, -55.4156) centre (-69.6121, -56.0156) ccw
  line L87 (-69.6121, -57.2156) -> (-97.0561, -57.2156)
  line L88 (-98.0954, -55.4156) -> (-84.3733, -31.6484)
  line L89 (-82.2949, -31.6484) -> (-68.5729, -55.4156)
  circle A39 centre (-68.2265, -56.8156) radius 0.4 construction
  line L90 (-68.5729, -56.6156) -> (-67.88, -57.0156) construction
  circle A40 centre (-66.6676, -57.7156) radius 3 construction
  line L91 (-83.3341, -57.7156) -> (-83.3341, -58.2156) construction
  line L92 (-68.5729, -56.6156) -> (-69.2657, -56.2156) construction
  line L93 (-83.3186, -28.8752) -> (-116.6516, -28.8752) construction
  line L94 (-116.6516, -28.8752) -> (-99.9851, -0.008) construction
  line L95 (-99.9851, -0.008) -> (-83.3186, -28.8752) construction
  line L96 (-84.1846, -28.3752) -> (-115.7856, -28.3752) construction
  line L97 (-115.7856, -28.3752) -> (-99.9851, -1.008) construction
  line L98 (-99.9851, -1.008) -> (-84.1846, -28.3752) construction
  line L99 (-99.9851, -28.3752) -> (-99.9851, -28.8752) construction
  line L100 (-107.8853, -14.6916) -> (-108.3184, -14.4416) construction
  line L101 (-92.0849, -14.6916) -> (-91.6519, -14.4416) construction
  arc A41 (-114.7464, -26.5752) -> (-113.7071, -28.3752) centre (-113.7071, -27.1752) ccw
  arc A42 (-98.9459, -2.808) -> (-101.0243, -2.808) centre (-99.9851, -3.408) ccw
  arc A43 (-86.2631, -28.3752) -> (-85.2239, -26.5752) centre (-86.2631, -27.1752) ccw
  line L102 (-86.2631, -28.3752) -> (-113.7071, -28.3752)
  line L103 (-114.7464, -26.5752) -> (-101.0243, -2.808)
  line L104 (-98.9459, -2.808) -> (-85.2239, -26.5752)
  circle A44 centre (-84.8775, -27.9752) radius 0.4 construction
  line L105 (-85.2239, -27.7752) -> (-84.531, -28.1752) construction
  circle A45 centre (-83.3186, -28.8752) radius 3 construction
  line L106 (-99.9851, -28.8752) -> (-99.9851, -29.3752) construction
  line L107 (-85.2239, -27.7752) -> (-85.9167, -27.3752) construction
  line L108 (-50.0011, -28.8484) -> (-83.3341, -28.8484) construction
  line L109 (-83.3341, -28.8484) -> (-66.6676, 0.0188) construction
  line L110 (-66.6676, 0.0188) -> (-50.0011, -28.8484) construction
  line L111 (-50.8671, -28.3484) -> (-82.4681, -28.3484) construction
  line L112 (-82.4681, -28.3484) -> (-66.6676, -0.9812) construction
  line L113 (-66.6676, -0.9812) -> (-50.8671, -28.3484) construction
  line L114 (-66.6676, -28.3484) -> (-66.6676, -28.8484) construction
  line L115 (-74.5678, -14.6648) -> (-75.0009, -14.4148) construction
  line L116 (-58.7674, -14.6648) -> (-58.3344, -14.4148) construction
  arc A46 (-81.4289, -26.5484) -> (-80.3896, -28.3484) centre (-80.3896, -27.1484) ccw
  arc A47 (-65.6284, -2.7812) -> (-67.7068, -2.7812) centre (-66.6676, -3.3812) ccw
  arc A48 (-52.9456, -28.3484) -> (-51.9064, -26.5484) centre (-52.9456, -27.1484) ccw
  line L117 (-52.9456, -28.3484) -> (-80.3896, -28.3484)
  line L118 (-81.4289, -26.5484) -> (-67.7068, -2.7812)
  line L119 (-65.6284, -2.7812) -> (-51.9064, -26.5484)
  circle A49 centre (-51.56, -27.9484) radius 0.4 construction
  line L120 (-51.9064, -27.7484) -> (-51.2135, -28.1484) construction
  circle A50 centre (-50.0011, -28.8484) radius 3 construction
  line L121 (-66.6676, -28.8484) -> (-66.6676, -29.3484) construction
  line L122 (-51.9064, -27.7484) -> (-52.5992, -27.3484) construction
  line L123 (-16.6681, -28.8484) -> (-50.0011, -28.8484) construction
  line L124 (-50.0011, -28.8484) -> (-33.3346, 0.0188) construction
  line L125 (-33.3346, 0.0188) -> (-16.6681, -28.8484) construction
  line L126 (-17.5341, -28.3484) -> (-49.1351, -28.3484) construction
  line L127 (-49.1351, -28.3484) -> (-33.3346, -0.9812) construction
  line L128 (-33.3346, -0.9812) -> (-17.5341, -28.3484) construction
  line L129 (-33.3346, -28.3484) -> (-33.3346, -28.8484) construction
  line L130 (-41.2348, -14.6648) -> (-41.6679, -14.4148) construction
  line L131 (-25.4344, -14.6648) -> (-25.0014, -14.4148) construction
  arc A51 (-48.0959, -26.5484) -> (-47.0566, -28.3484) centre (-47.0566, -27.1484) ccw
  arc A52 (-32.2954, -2.7812) -> (-34.3738, -2.7812) centre (-33.3346, -3.3812) ccw
  arc A53 (-19.6126, -28.3484) -> (-18.5734, -26.5484) centre (-19.6126, -27.1484) ccw
  line L132 (-19.6126, -28.3484) -> (-47.0566, -28.3484)
  line L133 (-48.0959, -26.5484) -> (-34.3738, -2.7812)
  line L134 (-32.2954, -2.7812) -> (-18.5734, -26.5484)
  circle A54 centre (-18.227, -27.9484) radius 0.4 construction
  line L135 (-18.5734, -27.7484) -> (-17.8805, -28.1484) construction
  circle A55 centre (-16.6681, -28.8484) radius 3 construction
  line L136 (-33.3346, -28.8484) -> (-33.3346, -29.3484) construction
  line L137 (-18.5734, -27.7484) -> (-19.2662, -27.3484) construction
  line L138 (-49.9979, -28.8484) -> (-16.6649, -28.8484) construction
  line L139 (-16.6649, -28.8484) -> (-33.3314, -57.7156) construction
  line L140 (-33.3314, -57.7156) -> (-49.9979, -28.8484) construction
  line L141 (-49.1319, -29.3484) -> (-17.5309, -29.3484) construction
  line L142 (-17.5309, -29.3484) -> (-33.3314, -56.7156) construction
  line L143 (-33.3314, -56.7156) -> (-49.1319, -29.3484) construction
  line L144 (-33.3314, -29.3484) -> (-33.3314, -28.8484) construction
  line L145 (-25.4312, -43.032) -> (-24.9981, -43.282) construction
  line L146 (-41.2316, -43.032) -> (-41.6646, -43.282) construction
  arc A56 (-18.5701, -31.1484) -> (-19.6094, -29.3484) centre (-19.6094, -30.5484) ccw
  arc A57 (-34.3706, -54.9156) -> (-32.2922, -54.9156) centre (-33.3314, -54.3156) ccw
  arc A58 (-47.0534, -29.3484) -> (-48.0926, -31.1484) centre (-47.0534, -30.5484) ccw
  line L147 (-47.0534, -29.3484) -> (-19.6094, -29.3484)
  line L148 (-18.5701, -31.1484) -> (-32.2922, -54.9156)
  line L149 (-34.3706, -54.9156) -> (-48.0926, -31.1484)
  circle A59 centre (-48.439, -29.7484) radius 0.4 construction
  line L150 (-48.0926, -29.9484) -> (-48.7855, -29.5484) construction
  circle A60 centre (-49.9979, -28.8484) radius 3 construction
  line L151 (-33.3314, -28.8484) -> (-33.3314, -28.3484) construction
  line L152 (-48.0926, -29.9484) -> (-47.3998, -30.3484) construction
  line L153 (-66.6676, 0.0188) -> (-33.3346, 0.0188) construction
  line L154 (-33.3346, 0.0188) -> (-50.0011, -28.8484) construction
  line L155 (-50.0011, -28.8484) -> (-66.6676, 0.0188) construction
  line L156 (-65.8016, -0.4812) -> (-34.2006, -0.4812) construction
  line L157 (-34.2006, -0.4812) -> (-50.0011, -27.8484) construction
  line L158 (-50.0011, -27.8484) -> (-65.8016, -0.4812) construction
  line L159 (-50.0011, -0.4812) -> (-50.0011, 0.0188) construction
  line L160 (-42.1009, -14.1648) -> (-41.6679, -14.4148) construction
  line L161 (-57.9013, -14.1648) -> (-58.3344, -14.4148) construction
  arc A61 (-35.2399, -2.2812) -> (-36.2791, -0.4812) centre (-36.2791, -1.6812) ccw
  arc A62 (-51.0403, -26.0484) -> (-48.9619, -26.0484) centre (-50.0011, -25.4484) ccw
  arc A63 (-63.7231, -0.4812) -> (-64.7624, -2.2812) centre (-63.7231, -1.6812) ccw
  line L162 (-63.7231, -0.4812) -> (-36.2791, -0.4812)
  line L163 (-35.2399, -2.2812) -> (-48.9619, -26.0484)
  line L164 (-51.0403, -26.0484) -> (-64.7624, -2.2812)
  circle A64 centre (-65.1088, -0.8812) radius 0.4 construction
  line L165 (-64.7624, -1.0812) -> (-65.4552, -0.6812) construction
  circle A65 centre (-66.6676, 0.0188) radius 3 construction
  line L166 (-50.0011, 0.0188) -> (-50.0011, 0.5188) construction
  line L167 (-64.7624, -1.0812) -> (-64.0695, -1.4812) construction
  line L168 (-33.3314, 0.0188) -> (0.0016, 0.0188) construction
  line L169 (0.0016, 0.0188) -> (-16.6649, -28.8484) construction
  line L170 (-16.6649, -28.8484) -> (-33.3314, 0.0188) construction
  line L171 (-32.4654, -0.4812) -> (-0.8644, -0.4812) construction
  line L172 (-0.8644, -0.4812) -> (-16.6649, -27.8484) construction
  line L173 (-16.6649, -27.8484) -> (-32.4654, -0.4812) construction
  line L174 (-16.6649, -0.4812) -> (-16.6649, 0.0188) construction
  line L175 (-8.7647, -14.1648) -> (-8.3316, -14.4148) construction
  line L176 (-24.5651, -14.1648) -> (-24.9981, -14.4148) construction
  arc A66 (-1.9036, -2.2812) -> (-2.9429, -0.4812) centre (-2.9429, -1.6812) ccw
  arc A67 (-17.7041, -26.0484) -> (-15.6257, -26.0484) centre (-16.6649, -25.4484) ccw
  arc A68 (-30.3869, -0.4812) -> (-31.4261, -2.2812) centre (-30.3869, -1.6812) ccw
  line L177 (-30.3869, -0.4812) -> (-2.9429, -0.4812)
  line L178 (-1.9036, -2.2812) -> (-15.6257, -26.0484)
  line L179 (-17.7041, -26.0484) -> (-31.4261, -2.2812)
  circle A69 centre (-31.7725, -0.8812) radius 0.4 construction
  line L180 (-31.4261, -1.0812) -> (-32.119, -0.6812) construction
  circle A70 centre (-33.3314, 0.0188) radius 3 construction
  line L181 (-16.6649, 0.0188) -> (-16.6649, 0.5188) construction
  line L182 (-31.4261, -1.0812) -> (-30.7333, -1.4812) construction
  line L183 (-83.317, -28.8188) -> (-49.984, -28.8188) construction
  line L184 (-49.984, -28.8188) -> (-66.6505, -57.686) construction
  line L185 (-66.6505, -57.686) -> (-83.317, -28.8188) construction
  line L186 (-82.451, -29.3188) -> (-50.85, -29.3188) construction
  line L187 (-50.85, -29.3188) -> (-66.6505, -56.686) construction
  line L188 (-66.6505, -56.686) -> (-82.451, -29.3188) construction
  line L189 (-66.6505, -29.3188) -> (-66.6505, -28.8188) construction
  line L190 (-58.7503, -43.0024) -> (-58.3173, -43.2524) construction
  line L191 (-74.5507, -43.0024) -> (-74.9838, -43.2524) construction
  arc A71 (-51.8893, -31.1188) -> (-52.9285, -29.3188) centre (-52.9285, -30.5188) ccw
  arc A72 (-67.6897, -54.886) -> (-65.6113, -54.886) centre (-66.6505, -54.286) ccw
  arc A73 (-80.3725, -29.3188) -> (-81.4117, -31.1188) centre (-80.3725, -30.5188) ccw
  line L192 (-80.3725, -29.3188) -> (-52.9285, -29.3188)
  line L193 (-51.8893, -31.1188) -> (-65.6113, -54.886)
  line L194 (-67.6897, -54.886) -> (-81.4117, -31.1188)
  circle A74 centre (-81.7582, -29.7188) radius 0.4 construction
  line L195 (-81.4117, -29.9188) -> (-82.1046, -29.5188) construction
  circle A75 centre (-83.317, -28.8188) radius 3 construction
  line L196 (-66.6505, -28.8188) -> (-66.6505, -28.3188) construction
  line L197 (-81.4117, -29.9188) -> (-80.7189, -30.3188) construction
  line L198 (-99.9974, 0.0188) -> (-66.6644, 0.0188) construction
  line L199 (-66.6644, 0.0188) -> (-83.3309, -28.8484) construction
  line L200 (-83.3309, -28.8484) -> (-99.9974, 0.0188) construction
  line L201 (-99.1314, -0.4812) -> (-67.5304, -0.4812) construction
  line L202 (-67.5304, -0.4812) -> (-83.3309, -27.8484) construction
  line L203 (-83.3309, -27.8484) -> (-99.1314, -0.4812) construction
  line L204 (-83.3309, -0.4812) -> (-83.3309, 0.0188) construction
  line L205 (-75.4307, -14.1648) -> (-74.9976, -14.4148) construction
  line L206 (-91.2311, -14.1648) -> (-91.6641, -14.4148) construction
  arc A76 (-68.5696, -2.2812) -> (-69.6089, -0.4812) centre (-69.6089, -1.6812) ccw
  arc A77 (-84.3701, -26.0484) -> (-82.2917, -26.0484) centre (-83.3309, -25.4484) ccw
  arc A78 (-97.0529, -0.4812) -> (-98.0921, -2.2812) centre (-97.0529, -1.6812) ccw
  line L207 (-97.0529, -0.4812) -> (-69.6089, -0.4812)
  line L208 (-68.5696, -2.2812) -> (-82.2917, -26.0484)
  line L209 (-84.3701, -26.0484) -> (-98.0921, -2.2812)
  circle A79 centre (-98.4385, -0.8812) radius 0.4 construction
  line L210 (-98.0921, -1.0812) -> (-98.785, -0.6812) construction
  circle A80 centre (-99.9974, 0.0188) radius 3 construction
  line L211 (-83.3309, 0.0188) -> (-83.3309, 0.5188) construction
  line L212 (-98.0921, -1.0812) -> (-97.3993, -1.4812) construction
  line L213 (-133.3304, -0.008) -> (-99.9974, -0.008) construction
  line L214 (-99.9974, -0.008) -> (-116.6639, -28.8752) construction
  line L215 (-116.6639, -28.8752) -> (-133.3304, -0.008) construction
  line L216 (-132.4644, -0.508) -> (-100.8634, -0.508) construction
  line L217 (-100.8634, -0.508) -> (-116.6639, -27.8752) construction
  line L218 (-116.6639, -27.8752) -> (-132.4644, -0.508) construction
  line L219 (-116.6639, -0.508) -> (-116.6639, -0.008) construction
  line L220 (-108.7637, -14.1916) -> (-108.3306, -14.4416) construction
  line L221 (-124.5641, -14.1916) -> (-124.9971, -14.4416) construction
  arc A81 (-101.9026, -2.308) -> (-102.9419, -0.508) centre (-102.9419, -1.708) ccw
  arc A82 (-117.7031, -26.0752) -> (-115.6247, -26.0752) centre (-116.6639, -25.4752) ccw
  arc A83 (-130.3859, -0.508) -> (-131.4251, -2.308) centre (-130.3859, -1.708) ccw
  line L222 (-130.3859, -0.508) -> (-102.9419, -0.508)
  line L223 (-101.9026, -2.308) -> (-115.6247, -26.0752)
  line L224 (-117.7031, -26.0752) -> (-131.4251, -2.308)
  circle A84 centre (-131.7715, -0.908) radius 0.4 construction
  line L225 (-131.4251, -1.108) -> (-132.118, -0.708) construction
  circle A85 centre (-133.3304, -0.008) radius 3 construction
  line L226 (-116.6639, -0.008) -> (-116.6639, 0.492) construction
  line L227 (-131.4251, -1.108) -> (-130.7323, -1.508) construction
  line L228 (-116.6671, -28.8484) -> (-83.3341, -28.8484) construction
  line L229 (-83.3341, -28.8484) -> (-100.0006, -57.7156) construction
  line L230 (-100.0006, -57.7156) -> (-116.6671, -28.8484) construction
  line L231 (-115.8011, -29.3484) -> (-84.2001, -29.3484) construction
  line L232 (-84.2001, -29.3484) -> (-100.0006, -56.7156) construction
  line L233 (-100.0006, -56.7156) -> (-115.8011, -29.3484) construction
  line L234 (-100.0006, -29.3484) -> (-100.0006, -28.8484) construction
  line L235 (-92.1004, -43.032) -> (-91.6674, -43.282) construction
  line L236 (-107.9008, -43.032) -> (-108.3339, -43.282) construction
  arc A86 (-85.2394, -31.1484) -> (-86.2786, -29.3484) centre (-86.2786, -30.5484) ccw
  arc A87 (-101.0398, -54.9156) -> (-98.9614, -54.9156) centre (-100.0006, -54.3156) ccw